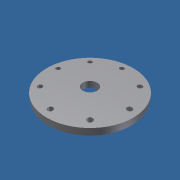
# Autodesk Inventor part: ServoFutabaS3003_circularArm
Saved by Autodesk Inventor 2012 (Build 160160000, 160)
## iProperties
Created: 2014-03-29
Part Number: ServoFutabaS3003_circularArm
Material: Default
Document SubType Name: Modeling
Designer: Admin
Density: 1 g/cm^3
Author: Admin
Autodesk Inventor part; units mm, degrees
ref_plane "YZ Plane" through (0, 0, 0) normal (1, 0, 0) x (0, 1, 0)
ref_plane "XZ Plane" through (0, 0, 0) normal (0, 1, 0) x (-1, 0, 0)
ref_plane "XY Plane" through (0, 0, 0) normal (0, 0, 1) x (1, 0, 0)
sketch "Sketch1" plane through (0, 0, 0) normal (0, 0, 1) x (1, 0, 0)
  circle A0 centre (0, 0) radius 17.8
  dimension "d0" = 35.6
  constraints: 1 centre point, 1 coincident
  measures "d0" diameter of A0
extrude "Extrusion1" add sketch "Sketch1" along normal blind 2.54
sketch "Sketch2" plane through (0, 0, 2.54) normal (0, 0, 1) x (1, 0, 0)
  circle A0 centre (0, 0) radius 17.8 projected
  line L0 (-24.92, 0) -> (24.92, 0) projected
  line L1 (0, -24.92) -> (0, 24.92) projected
  circle A1 centre (0, 14.84) radius 1
  circle A2 centre (-10.4935, 10.4935) radius 1
  circle A3 centre (-14.84, 0) radius 1
  circle A4 centre (-10.4935, -10.4935) radius 1
  circle A5 centre (0, -14.84) radius 1
  circle A6 centre (10.4935, -10.4935) radius 1
  circle A7 centre (14.84, 0) radius 1
  circle A8 centre (10.4935, 10.4935) radius 1
  circle A9 centre (0, 0) radius 3
  dimension "d3" = 2
  dimension "d4" = 14.84
  dimension "d7" = 360
  dimension "d9" = 6
  constraints: 9 centre point, 1 coincident, 1 point on line, 17 other
  measures "d3" diameter of A1
  measures "d4" distance from line of L0 A1.centre
  measures "d9" diameter of A9
extrude "Extrusion2" cut sketch "Sketch2" against normal blind 2.54 contours A7 L0 | L0 A7 | A1 L1 | L1 A1 | A5 L1 | L1 A5 | A3 L0 | L0 A3 | A9 L1 L0 | L0 L1 A9 | L1 L0 A9 | A9 L0 L1 | A2 | A4 | A6 | A8
body "Solid1"
